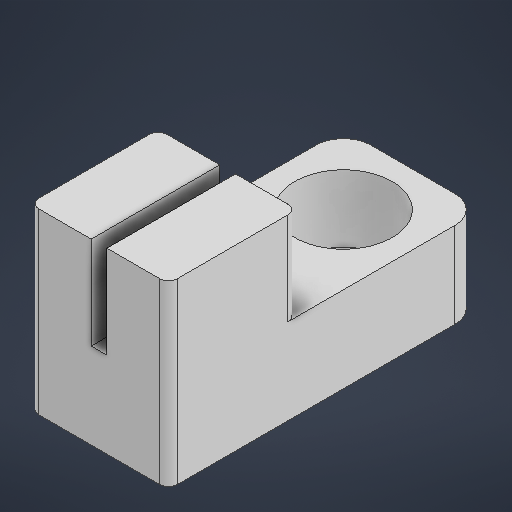
# Autodesk Inventor part: Solderaid
Saved by Autodesk Inventor 2025 (Build 290162010, 162A)
## iProperties
Created: 2025-03-10
Part Number: Solderaid
Material: Generic
Document SubType Name: Modeling
Designer: tzu98
Density: 1 g/cm^3
Appearance: Default
Author: tzu98
Autodesk Inventor part; units mm, degrees
ref_plane "YZ Plane" through (0, 0, 0) normal (1, 0, 0) x (0, 1, 0)
ref_plane "XZ Plane" through (0, 0, 0) normal (0, 1, 0) x (-1, 0, 0)
ref_plane "XY Plane" through (0, 0, 0) normal (0, 0, 1) x (1, 0, 0)
sketch "Sketch1" plane through (0, 0, 0) normal (0, 0, 1) x (1, 0, 0)
  line L0 (-7.5, 16.9418) -> (7.5, 16.9418)
  line L1 (7.5, 16.9418) -> (7.5, -16.9418)
  line L2 (7.5, -16.9418) -> (-7.5, -16.9418)
  line L3 (-7.5, -16.9418) -> (-7.5, 16.9418)
  line L4 (-7.5, 16.9418) -> (7.5, -16.9418) construction
  line L5 (7.5, 16.9418) -> (-7.5, -16.9418) construction
  circle A0 centre (0, 9.4418) radius 5.25
  point P0 (0, 0)
  dimension "d0" = 10.5
  dimension "d1" = 7.5
  dimension "d2" = 15
  constraints: 12 end point, 2 midpoint, 2 parallel, 1 centre point, 1 horizontal, 1 perpendicular
  measures "d0" diameter of A0
  measures "d1" distance from line of L0 A0.centre
  measures "d2" distance between parallel lines of L3 L1
extrude "Extrusion1" add sketch "Sketch1" along normal blind 7.25
fillet "Fillet1" radius 3 2 edges at (7.5, 16.9418, 3.625) (-7.5, 16.9418, 3.625)
sketch "Sketch2" plane through (0, 0, 0) normal (0, 0, -1) x (-1, 0, 0)
  arc A0 (7.5, 13.9418) -> (4.5, 16.9418) centre (4.5, 13.9418) ccw projected
  line L0 (-4.5, 16.9418) -> (4.5, 16.9418) projected
  arc A1 (-4.5, 16.9418) -> (-7.5, 13.9418) centre (-4.5, 13.9418) ccw projected
  line L1 (-7.5, -16.9418) -> (-7.5, 13.9418) projected
  line L2 (7.5, -16.9418) -> (-7.5, -16.9418) projected
  line L3 (7.5, 13.9418) -> (7.5, -16.9418) projected
  circle A2 centre (0, 9.4418) radius 5.25 projected
  circle A3 centre (0, 9.4418) radius 4
  point P0 (0, 0)
  dimension "d6" = 8
  constraints: 1 centre point, 1 coincident
  measures "d6" diameter of A3
extrude "Extrusion2" add sketch "Sketch2" along normal blind 2 contours L3 L2 L1 A1 L0 A0 | A2
sketch "Sketch3" plane through (0, 0, 7.25) normal (0, 0, 1) x (1, 0, 0)
  line L0 (-7.5, -16.9418) -> (7.5, -16.9418) projected
  line L1 (-7.5, -16.9418) -> (-0.85, -16.9418)
  line L2 (-0.85, -16.9418) -> (-0.85, -3.0582)
  line L3 (-0.85, -3.0582) -> (-7.5, -3.0582)
  line L4 (-7.5, -3.0582) -> (-7.5, -16.9418)
  line L5 (7.5, -3.0582) -> (0.85, -3.0582)
  line L6 (0.85, -3.0582) -> (0.85, -16.9418)
  line L7 (0.85, -16.9418) -> (7.5, -16.9418)
  line L8 (7.5, -16.9418) -> (7.5, -3.0582)
  line L9 (4.5, 16.9418) -> (-4.5, 16.9418) projected
  point P0 (0, 0)
  point P1 (-0.85, -16.9418)
  dimension "d10" = 0.85
  dimension "d11" = 0.85
  dimension "d12" = 20
  constraints: 16 end point, 4 parallel, 2 horizontal, 2 perpendicular, 2 point on line
  measures "d10" distance from line of point (0, 0) L6
  measures "d11" distance from line of L2 point (0, 0)
  measures "d12" distance between parallel lines of L9 L5
extrude "Extrusion3" add sketch "Sketch3" along normal blind 10
fillet "Fillet2" radius 1 4 edges at (7.5, -3.0582, 12.25) (7.5, -16.9418, 7.625) (-7.5, -16.9418, 7.625) (-7.5, -3.0582, 12.25)
body "Solid1"
